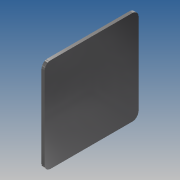
# Autodesk Inventor part: DD_KVD_003_09_B
Saved by Autodesk Inventor 2017.3 (Build 213256000, 256)
## iProperties
Created: 2023-12-04
Part Number: DD_KVD_003_09_B
Material: Nerezová ocel
Document SubType Name: Sheet Metal
Designer: Darena
Density: 8 g/cm^3
Flat Pattern Width: 9.1 cm
Flat Pattern Length: 9.1 cm
Flat Pattern Area: 82.81 cm^2
Sheet Metal Rule: Výchozí_mm
Sheet Metal Width: 91,000 mm
Sheet Metal Length: 91,000 mm
Sheet Metal Area: 8281,000 mm^2
Appearance: Pololeštěná
Author: Darena
Title: DÍL SVAŘENCE - 08
Autodesk Inventor part; units mm, degrees
ref_plane "YZ Plane" through (0, 0, 0) normal (1, 0, 0) x (0, 1, 0)
ref_plane "XZ Plane" through (0, 0, 0) normal (0, 1, 0) x (-1, 0, 0)
ref_plane "XY Plane" through (0, 0, 0) normal (0, 0, 1) x (1, 0, 0)
sketch "Náčrt2" plane through (0, 0, 0) normal (1, 0, 0) x (0, 1, 0)
  line L0 (45.5, 45.5) -> (-45.5, 45.5)
  line L1 (-45.5, -45.5) -> (45.5, -45.5)
  line L2 (45.5, -45.5) -> (45.5, 45.5)
  line L3 (-45.5, 45.5) -> (-45.5, -45.5)
  point P0 (-45.5, 0)
  point P1 (0, 0)
  point P2 (0, 45.5)
  dimension "d1" = 91
  dimension "d62" = 91
  constraints: 8 end point, 2 midpoint, 1 horizontal, 1 horizontal alignment, 1 parallel, 1 perpendicular, 1 vertical, 1 vertical alignment
  measures "d1" distance of L0.start L0.end
  measures "d62" distance of L0.end L1.start
extrude "Vysunutí1" add sketch "Náčrt2" against normal blind 3
fillet "Zaoblení1" radius 6 4 edges at (-1.5, -45.5, -45.5) (-1.5, 45.5, -45.5) (-1.5, -45.5, 45.5) (-1.5, 45.5, 45.5)
equation "\"d62\" = d1"
equation "\"PoloměrOhybu\" = Tloušťka"
equation "\"ŠířkaVýštipu\" = Tloušťka"
equation "\"HloubkaVýštipu\" = 0.5 * Tloušťka"
equation "\"VelikostRohovéhoVýštipu\" = 4 * Tloušťka"
equation "\"MinimálníZbytek\" = 2 * Tloušťka"
equation "\"PřechodovýPoloměr\" = PoloměrOhybu"
equation "\"VelikostJacobihoPoloměru\" = PoloměrOhybu"
equation "\"VelikostMezery\" = Tloušťka"
equation "\"Tloušťka\" = 3"
